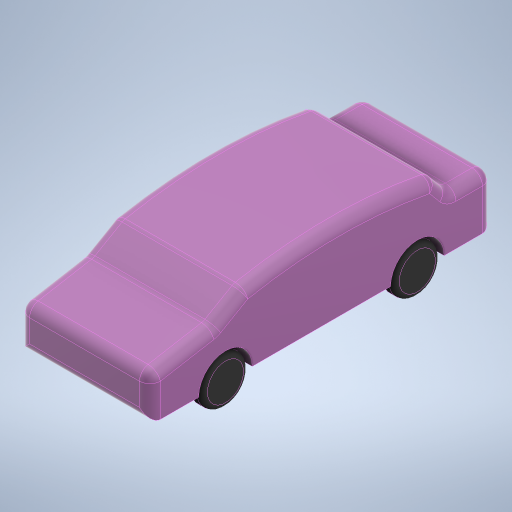
# Autodesk Inventor part: BungaCamp-Sedan
Saved by Autodesk Inventor 2023 (Build 270158000, 158)
## iProperties
Created: 2024-07-15
Part Number: BungaCamp-Sedan
Material: Generic
Document SubType Name: Modeling
Designer: incep
Density: 1 g/cm^3
Appearance: Smooth - Purple
Author: incep
Autodesk Inventor part; units mm, degrees
ref_plane "YZ Plane" through (0, 0, 0) normal (1, 0, 0) x (0, 1, 0)
ref_plane "XZ Plane" through (0, 0, 0) normal (0, 1, 0) x (-1, 0, 0)
ref_plane "XY Plane" through (0, 0, 0) normal (0, 0, 1) x (1, 0, 0)
sketch "Sketch1" plane through (0, 0, 0) normal (1, 0, 0) x (0, 1, 0)
  line L0 (600, 2457.5) -> (0, 2457.5)
  line L1 (0, 2457.5) -> (0, -2457.5)
  circle A0 centre (0, 1375) radius 334.35
  circle A1 centre (0, -1375) radius 334.35
  line L2 (0, 1375) -> (0, -1375) construction
  line L3 (761.3392, 1542.5) -> (1011.4126, 1109.3602)
  line L4 (1011.4126, 1109.3602) -> (1011.4126, -1629.7578)
  line L5 (1011.4126, -1629.7578) -> (740, -1857.5)
  line L6 (740, -1857.5) -> (740, -2457.5)
  line L7 (-334.35, -1040.65) -> (-334.35, -1709.35) construction
  line L8 (600, 2457.5) -> (761.3392, 1542.5)
  line L9 (0, -2457.5) -> (740, -2457.5)
  circle A2 centre (0, 1375) radius 384.35
  circle A3 centre (0, -1375) radius 384.35
  arc A4 (1011.4126, -1629.7578) -> (1011.4126, 1109.3602) centre (-5907.94, -260.1988) ccw
  line L10 (1145.65, 637.3331) -> (1145.65, -1157.7308) construction
  point P0 (0, 0)
  point P1 (0, 0)
  point P2 (-334.35, -1375)
  point P3 (0, 1759.35)
  point P4 (0, 990.65)
  point P5 (0, -990.65)
  point P6 (0, -1759.35)
  point P7 (1145.65, -260.1988)
  dimension "d0" = 668.7
  dimension "d1" = 2750
  dimension "d2" = 4915
  dimension "d4" = 50
  dimension "d5" = 50
  dimension "d6" = 100
  dimension "d7" = 150
  dimension "d8" = 915
  dimension "d9" = 600
  dimension "d10" = 740
  dimension "d11" = 130
  dimension "d12" = 600
  dimension "d22" = 1480
  constraints: 22 end point, 5 centre point, 4 midpoint, 3 point on circle, 3 vertical, 2 horizontal, 2 point on line, 1 coincident, 1 collinear, 1 equal radius, 1 horizontal alignment, 1 parallel, 1 perpendicular, 1 tangent
  measures "d0" diameter of A0
  measures "d1" distance of L2.end L2.start
  measures "d2" distance of L0.end L1.end
  measures "d4" radial gap between concentric circles of A0 A2
  measures "d5" radial gap between concentric circles of A1 A3
  measures "d6" angle of L8 L0
  measures "d7" angle of L4 L3
  measures "d8" distance from line of L0 L3.start
  measures "d9" distance of L0.start L0.end
  measures "d10" distance of L1.end L6.end
  measures "d11" angle of L4 L5
  measures "d12" distance of L5.end L6.end
  measures "d22" distance between parallel lines of L7 L10
extrude "Extrusion1" add sketch "Sketch1" along normal mid plane 1875 contours L8 L3 L4 L5 L6 L9 L1 A3 A2 L0 | A4 L4
sketch "Sketch2" plane through (937.5, 0, 0) normal (1, 0, 0) x (0, 0, -1)
  circle A0 centre (-1375, 0) radius 334.35 projected
  circle A1 centre (1375, 0) radius 334.35 projected
  point P0 (0, 0)
extrude "Extrusion2" add sketch "Sketch2" against normal blind 235
sketch "Sketch3" plane through (-937.5, 0, 0) normal (-1, 0, 0) x (0, 0, 1)
  circle A0 centre (-1375, 0) radius 334.35 projected
  circle A1 centre (1375, 0) radius 334.35 projected
  point P0 (0, 0)
extrude "Extrusion3" add sketch "Sketch3" against normal blind 235
fillet "Fillet1" radius 150 22 edges at (0, 740, -2457.5) (0, 740, -1857.5) (0, 1011.4126, -1629.7578) (0, 1011.4126, 1109.3602) (0, 761.3392, 1542.5) (0, 600, 2457.5) (0, 0, 2457.5) (-937.5, 300, 2457.5) (937.5, 300, 2457.5) (-937.5, 680.6696, 2000) (-937.5, 886.3759, 1325.9301) (937.5, 886.3759, 1325.9301) (937.5, 680.6696, 2000) (-937.5, 740, -2157.5) (937.5, 875.7063, -1743.6289) (937.5, 740, -2157.5) (937.5, 370, -2457.5) (0, 0, -2457.5) (-937.5, 370, -2457.5) (-937.5, 875.7063, -1743.6289) (937.5, 1145.65, -260.1988) (-937.5, 1145.65, -260.1988)
fillet "Fillet2" radius 75 8 edges at (937.5, 0, 1709.35) (937.5, 0, -1040.65) (702.5, 0, -1040.65) (702.5, 0, 1709.35) (-702.5, 0, 1040.65) (-937.5, 0, 1040.65) (-702.5, 0, -1709.35) (-937.5, 0, -1709.35)
body "Solid1"
